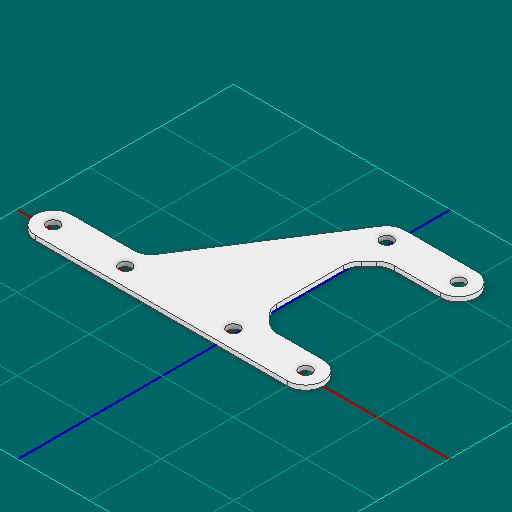
# Autodesk Inventor part: gusset
Saved by Autodesk Inventor 2025 (Build 290162000, 162)
## iProperties
Created: 2024-08-19
Part Number: gusset
Material: Acetal Resin, White
Document SubType Name: Modeling
Designer: averey
Density: 1.425 g/cm^3
Appearance: Smooth - White
Author: averey
Autodesk Inventor part; units mm, degrees
ref_plane "YZ Plane" through (0, 0, 0) normal (1, 0, 0) x (0, 1, 0)
ref_plane "XZ Plane" through (0, 0, 0) normal (0, 1, 0) x (-1, 0, 0)
ref_plane "XY Plane" through (0, 0, 0) normal (0, 0, 1) x (1, 0, 0)
sketch "main" plane through (0, 0, 0) normal (0, 0, 1) x (1, 0, 0)
  circle A0 centre (-18.4512, -23.1863) radius 2.1844
  line L0 (-22.9413, -14.9764) -> (-20.311, -12.3462)
  line L1 (-43.8512, -16.8363) -> (-27.4314, -16.8363)
  arc A1 (-27.4314, -16.8363) -> (-22.9413, -14.9764) centre (-27.4314, -10.4863) ccw
  circle A2 centre (-43.8512, -23.1863) radius 2.1844
  arc A3 (-43.8512, -16.8363) -> (-43.8512, -29.5363) centre (-43.8512, -23.1863) ccw
  arc A4 (-20.311, -12.3462) -> (-18.4512, -7.856) centre (-24.8012, -7.856) ccw
  line L2 (-18.4512, 15.4585) -> (-18.4512, -7.856)
  line L3 (17.7748, 21.5177) -> (-13.1066, -26.6153)
  arc A5 (-18.4512, 15.4585) -> (-20.311, 19.9486) centre (-24.8012, 15.4585) ccw
  line L4 (-22.9413, 22.5788) -> (-20.311, 19.9486)
  arc A6 (-22.9413, 22.5788) -> (-27.4314, 24.4387) centre (-27.4314, 18.0887) ccw
  circle A7 centre (-43.8512, 30.7887) radius 2.1844
  circle A8 centre (-18.4512, 30.7887) radius 2.1844
  circle A9 centre (19.6488, 30.7887) radius 2.1844
  line L5 (45.0488, 37.1387) -> (-43.8512, 37.1387)
  line L6 (-27.4314, 24.4387) -> (-43.8512, 24.4387)
  arc A10 (-43.8512, 37.1387) -> (-43.8512, 24.4387) centre (-43.8512, 30.7887) ccw
  arc A11 (23.1193, 24.4387) -> (17.7748, 21.5177) centre (23.1193, 18.0887) ccw
  line L7 (45.0488, 24.4387) -> (23.1193, 24.4387)
  circle A12 centre (45.0488, 30.7887) radius 2.1844
  arc A13 (45.0488, 24.4387) -> (45.0488, 37.1387) centre (45.0488, 30.7887) ccw
  line L8 (-18.4512, -29.5363) -> (-43.8512, -29.5363)
  arc A14 (-18.4512, -29.5363) -> (-13.1066, -26.6153) centre (-18.4512, -23.1863) ccw
  point P0 (-14.0637, 6.8091)
  dimension "d0" = 6.35
  dimension "d1" = 6.35
  measures "d0" radius of A11
  measures "d1" radius of A6
sketch "Sketch1" plane through (0, 0, 0) normal (0, 1, 0) x (-1, 0, 0)
  circle A0 centre (0, -53.975) radius 2.1844
  line L0 (-4.4901, -45.7651) -> (-1.8599, -43.1349)
  line L1 (-25.4, -47.625) -> (-8.9803, -47.625)
  arc A1 (-8.9803, -47.625) -> (-4.4901, -45.7651) centre (-8.9803, -41.275) ccw
  circle A2 centre (-25.4, -53.975) radius 2.1844
  arc A3 (-25.4, -47.625) -> (-25.4, -60.325) centre (-25.4, -53.975) ccw
  arc A4 (-1.8599, -43.1349) -> (0, -38.6447) centre (-6.35, -38.6447) ccw
  line L2 (0, -15.3303) -> (0, -38.6447)
  line L3 (36.2259, -9.271) -> (5.3446, -57.404)
  arc A5 (0, -15.3303) -> (-1.8599, -10.8401) centre (-6.35, -15.3303) ccw
  line L4 (-4.4901, -8.2099) -> (-1.8599, -10.8401)
  arc A6 (-4.4901, -8.2099) -> (-8.9803, -6.35) centre (-8.9803, -12.7) ccw
  circle A7 centre (-25.4, 0) radius 2.1844
  circle A8 centre (0, 0) radius 2.1844
  circle A9 centre (38.1, 0) radius 2.1844
  line L5 (63.5, 6.35) -> (-25.4, 6.35)
  line L6 (-8.9803, -6.35) -> (-25.4, -6.35)
  arc A10 (-25.4, 6.35) -> (-25.4, -6.35) centre (-25.4, 0) ccw
  arc A11 (41.5705, -6.35) -> (36.2259, -9.271) centre (41.5705, -12.7) ccw
  line L7 (63.5, -6.35) -> (41.5705, -6.35)
  circle A12 centre (63.5, 0) radius 2.1844
  arc A13 (63.5, -6.35) -> (63.5, 6.35) centre (63.5, 0) ccw
  line L8 (0, -60.325) -> (-25.4, -60.325)
  arc A14 (0, -60.325) -> (5.3446, -57.404) centre (0, -53.975) ccw
  constraints: 1 other
extrude "Extrusion1" add sketch "Sketch1" along normal blind 1.5875
body "Solid1"
